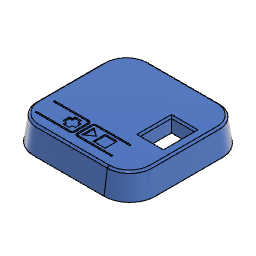
Abdeckung (Autodesk Fusion 360 design; units mm, degrees)
Autodesk Fusion 360 part; units mm, degrees
ref_plane "Arbeitsebene1" through (35.3452, 7.7218, 7.3701) normal (0, 0, 1) x (1, 0, 0)
sketch "Skizze1" plane through (35.3452, 7.7218, 7.3701) normal (0, 0, 1) x (1, 0, 0)
  line L0 (-56.34, -21.7733) -> (-56.34, 68.7267)
  arc A0 (-56.34, -21.7733) -> (-41.34, -36.7733) centre (-41.34, -21.7733) ccw
  line L1 (-0.34, -36.7733) -> (-41.34, -36.7733)
  arc A1 (-0.34, -36.7733) -> (14.66, -21.7733) centre (-0.34, -21.7733) ccw
  line L2 (14.66, 68.7267) -> (14.66, -21.7733)
  line L3 (12.66, 17.2267) -> (12.66, -21.7733)
  arc A2 (-0.34, -34.7733) -> (12.66, -21.7733) centre (-0.34, -21.7733) ccw
  line L4 (-0.34, -34.7733) -> (-41.34, -34.7733)
  arc A3 (-54.34, -21.7733) -> (-41.34, -34.7733) centre (-41.34, -21.7733) ccw
  line L5 (-54.34, -21.7733) -> (-54.34, 17.2267)
  line L6 (-41.34, 30.2267) -> (-0.34, 30.2267)
  circle A4 centre (-20.84, -2.2733) radius 32.5
  arc A5 (-41.34, 30.2267) -> (-54.34, 17.2267) centre (-41.34, 17.2267) ccw
  arc A6 (12.66, 17.2267) -> (-0.34, 30.2267) centre (-0.34, 17.2267) ccw
  dimension "d140" = 13
  dimension "d141" = 13
  constraint perpendicular L3 L6
  constraint tangent L6 A4
  constraint parallel L2 L3
  constraint concentric A1 A2
  constraint parallel L1 L4
  constraint concentric A0 A3
  constraint parallel L0 L5
  constraint tangent L4 A3
  constraint tangent L3 A2
  constraint tangent A2 L4
  constraint tangent A3 L5
  constraint tangent L5 A5
  constraint tangent L6 A5
  constraint tangent L4 A4
  constraint tangent L6 A6
  constraint tangent L3 A6
  measures "d140" radius of A5
  measures "d141" radius of A6
sketch "Skizze3" plane through (0, 0, -6.9849) normal (0, 0, 1) x (-1, 0, 0)
  circle A0 centre (-14.5052, -5.4485) radius 32.5
  circle A1 centre (-14.5052, -63.9485) radius 21.5
  arc A2 (-35.0052, 29.0515) -> (-50.0052, 14.0515) centre (-35.0052, 14.0515) ccw
  line L0 (-50.0052, 14.0515) -> (-50.0052, -76.4485)
  arc A3 (-50.0052, -76.4485) -> (-35.0052, -91.4485) centre (-35.0052, -76.4485) ccw
  line L1 (-35.0052, -91.4485) -> (5.9948, -91.4485)
  arc A4 (5.9948, -91.4485) -> (20.9948, -76.4485) centre (5.9948, -76.4485) ccw
  line L2 (20.9948, -76.4485) -> (20.9948, 14.0515)
  arc A5 (20.9948, 14.0515) -> (5.9948, 29.0515) centre (5.9948, 14.0515) ccw
  line L3 (5.9948, 29.0515) -> (-35.0052, 29.0515)
  arc A6 (20.9948, 14.0515) -> (5.9948, 29.0515) centre (5.9948, 14.0515) ccw
  line L4 (-35.0052, 29.0515) -> (5.9948, 29.0515)
  arc A7 (-35.0052, 29.0515) -> (-50.0052, 14.0515) centre (-35.0052, 14.0515) ccw
  line L5 (-50.0052, -76.4485) -> (-50.0052, 14.0515)
  line L6 (20.9948, 14.0515) -> (20.9948, -76.4485)
  line L7 (5.9948, -39.9485) -> (-35.0052, -39.9485)
  arc A8 (5.9948, -39.9485) -> (20.9607, -23.9379) centre (5.9948, -24.9485) ccw
  arc A9 (-50.0052, -24.9485) -> (-35.0052, -39.9485) centre (-35.0052, -24.9485) ccw
  arc A10 (5.9948, -37.9485) -> (18.9948, -24.9485) centre (5.9948, -24.9485) ccw
  constraint perpendicular L0 L7
  constraint tangent L2 A8
  constraint tangent L5 A9
  constraint tangent L7 A8
  constraint tangent L7 A9
  constraint equal A8 A9
  constraint concentric A8 A10
  constraint coincident L5 A9.start
loft "Erhebung1" add profiles "Skizze3", "Skizze1" section 1 contours A2 L0 L2 A5 L3 A6 L4 A7 L5 L6 L7 A8 A9 section 2
sketch "Skizze4" plane through (0, 0, -6.9849) normal (0, 0, -1) x (1, 0, 0)
  spline S0 degree 3 poles (35.0052, 29.0515) (36.8795, 29.0515) (38.8639, 28.6884) (40.741, 27.9116) (42.1372, 27.3338) (43.4713, 26.5301) (44.6549, 25.5356) (46.3943, 24.074) (47.7962, 22.1974) (48.704, 20.1624) (49.5899, 18.1766) (50.0052, 16.0511) (50.0052, 14.0515) (50.0052, 1.0515) (50.0052, -11.9485) (50.0052, -24.9485) (50.0052, -26.8227) (49.6421, -28.8072) (48.8653, -30.6842) (48.2875, -32.0805) (47.4838, -33.4146) (46.4893, -34.5981) (45.0277, -36.3376) (43.1511, -37.7395) (41.1162, -38.6473) (39.1303, -39.5331) (37.0049, -39.9485) (35.0052, -39.9485) (21.3386, -39.9485) (7.6719, -39.9485) (-5.9948, -39.9485) (-7.869, -39.9485) (-9.8534, -39.5853) (-11.7305, -38.8085) (-13.1268, -38.2307) (-14.4609, -37.4271) (-15.6444, -36.4326) (-17.3839, -34.971) (-18.7858, -33.0943) (-19.6935, -31.0594) (-20.5794, -29.0736) (-20.9948, -26.9481) (-20.9948, -24.9485) (-20.9948, -11.9485) (-20.9948, 1.0515) (-20.9948, 14.0515) (-20.9948, 15.9258) (-20.6316, 17.9102) (-19.8548, 19.7872) (-19.277, 21.1835) (-18.4733, 22.5176) (-17.4789, 23.7011) (-16.0173, 25.4406) (-14.1406, 26.8425) (-12.1057, 27.7503) (-10.1199, 28.6362) (-7.9944, 29.0515) (-5.9948, 29.0515) (7.6719, 29.0515) (21.3386, 29.0515) (35.0052, 29.0515) knots 0 0 0 0 0.02269 0.02269 0.02269 0.039568 0.039568 0.039568 0.064375 0.064375 0.064375 0.088583 0.088583 0.088583 0.245965 0.245965 0.245965 0.268655 0.268655 0.268655 0.285533 0.285533 0.285533 0.31034 0.31034 0.31034 0.334548 0.334548 0.334548 0.5 0.5 0.5 0.52269 0.52269 0.52269 0.539568 0.539568 0.539568 0.564375 0.564375 0.564375 0.588583 0.588583 0.588583 0.745965 0.745965 0.745965 0.768655 0.768655 0.768655 0.785533 0.785533 0.785533 0.81034 0.81034 0.81034 0.834548 0.834548 0.834548 1 1 1 1
  circle A0 centre (14.5052, -5.4485) radius 32.5
extrude "Extrusion1" cut sketch "Skizze4" against normal blind 12 contours A0
sketch "Skizze5" plane through (0, 0, 7.3701) normal (0, 0, 1) x (-1, 0, 0)
  spline S0 degree 3 poles (-35.0052, 27.0515) (-36.7488, 27.0515) (-38.4915, 26.6961) (-40.0958, 26.0134) (-41.2892, 25.5055) (-42.4058, 24.8178) (-43.3964, 23.9807) (-44.8523, 22.7503) (-46.0324, 21.1954) (-46.8257, 19.4622) (-47.6, 17.7708) (-48.0052, 15.9117) (-48.0052, 14.0515) (-48.0052, 1.9582) (-48.0052, -12.8552) (-48.0052, -24.9485) (-48.0052, -26.692) (-47.6498, -28.4348) (-46.9671, -30.0391) (-46.4592, -31.2324) (-45.7716, -32.3491) (-44.9344, -33.3396) (-43.704, -34.7955) (-42.1491, -35.9756) (-40.4159, -36.769) (-38.7245, -37.5432) (-36.8654, -37.9485) (-35.0052, -37.9485) (-22.2917, -37.9485) (-6.7187, -37.9485) (5.9948, -37.9485) (7.7383, -37.9485) (9.481, -37.5931) (11.0853, -36.9103) (12.2787, -36.4025) (13.3953, -35.7148) (14.3859, -34.8777) (15.8418, -33.6473) (17.0219, -32.0924) (17.8153, -30.3592) (18.5895, -28.6678) (18.9948, -26.8087) (18.9948, -24.9485) (18.9948, -12.8552) (18.9948, 1.9582) (18.9948, 14.0515) (18.9948, 15.795) (18.6394, 17.5378) (17.9566, 19.1421) (17.4488, 20.3354) (16.7611, 21.4521) (15.924, 22.4427) (14.6936, 23.8986) (13.1387, 25.0787) (11.4054, 25.872) (9.7141, 26.6462) (7.8549, 27.0515) (5.9948, 27.0515) (-6.7187, 27.0515) (-22.2917, 27.0515) (-35.0052, 27.0515) knots 0 0 0 0 0.02269 0.02269 0.02269 0.039568 0.039568 0.039568 0.064375 0.064375 0.064375 0.088583 0.088583 0.088583 0.245965 0.245965 0.245965 0.268655 0.268655 0.268655 0.285533 0.285533 0.285533 0.31034 0.31034 0.31034 0.334548 0.334548 0.334548 0.5 0.5 0.5 0.52269 0.52269 0.52269 0.539568 0.539568 0.539568 0.564375 0.564375 0.564375 0.588583 0.588583 0.588583 0.745965 0.745965 0.745965 0.768655 0.768655 0.768655 0.785533 0.785533 0.785533 0.81034 0.81034 0.81034 0.834548 0.834548 0.834548 1 1 1 1
  line L0 (-41.6202, -16.3468) -> (-29.0702, -16.3468)
  line L1 (-29.0702, -16.3468) -> (-29.0702, 0.9032)
  line L2 (-29.0702, 0.9032) -> (-41.6202, 0.9032)
  line L3 (-41.6202, 0.9032) -> (-41.6202, -16.3468)
  line L4 (-33.512, -14.2079) -> (-33.069, -14.7358)
  line L5 (-33.069, -14.7358) -> (-33.4529, -15.0579)
  line L6 (-33.4529, -15.0579) -> (-39.8251, -15.0579)
  line L7 (-39.8251, -15.0579) -> (-40.0801, -14.7541)
  line L8 (-40.0801, -14.7541) -> (-39.4292, -14.2079)
  line L9 (-39.4292, -14.2079) -> (-33.512, -14.2079)
  line L10 (-39.6216, -13.9781) -> (-40.2727, -14.5245)
  line L11 (-40.2727, -14.5245) -> (-40.5275, -14.2209)
  line L12 (-40.5275, -14.2209) -> (-39.4684, -8.2142)
  line L13 (-39.4684, -8.2142) -> (-38.976, -7.8695)
  line L14 (-38.976, -7.8695) -> (-38.6313, -8.3618)
  line L15 (-38.6313, -8.3618) -> (-39.6216, -13.9781)
  line L16 (-39.2687, -7.0817) -> (-38.3065, -1.625)
  line L17 (-38.3065, -1.625) -> (-37.9226, -1.3029)
  line L18 (-37.9226, -1.3029) -> (-37.9169, -1.3098)
  line L19 (-37.9169, -1.3098) -> (-37.4797, -1.8308)
  line L20 (-37.4797, -1.8308) -> (-38.4316, -7.2293)
  line L21 (-38.4316, -7.2293) -> (-38.924, -7.5741)
  line L22 (-38.924, -7.5741) -> (-39.2687, -7.0817)
  circle A0 centre (-39.5952, -1.6629) radius 0.875
  line L23 (-31.1397, -1.8673) -> (-30.4891, -1.3214)
  line L24 (-30.4891, -1.3214) -> (-30.234, -1.6255)
  line L25 (-30.234, -1.6255) -> (-31.2221, -7.2293)
  line L26 (-31.2221, -7.2293) -> (-31.7144, -7.5741)
  line L27 (-31.7144, -7.5741) -> (-32.0592, -7.0817)
  line L28 (-32.0592, -7.0817) -> (-31.1397, -1.8673)
  line L29 (-32.133, -7.5003) -> (-32.1322, -7.5004)
  line L30 (-32.1322, -7.5004) -> (-32.0106, -7.6742)
  line L31 (-32.0106, -7.6742) -> (-32.1843, -7.7958)
  line L32 (-32.1843, -7.7958) -> (-32.1851, -7.7957)
  line L33 (-32.1851, -7.7957) -> (-32.1852, -7.7964)
  line L34 (-32.1852, -7.7964) -> (-32.6855, -8.1468)
  line L35 (-32.6855, -8.1468) -> (-38.4157, -8.1468)
  line L36 (-38.4157, -8.1468) -> (-38.5576, -7.944)
  line L37 (-38.5576, -7.944) -> (-38.5575, -7.9433)
  line L38 (-38.5575, -7.9433) -> (-38.5582, -7.9432)
  line L39 (-38.5582, -7.9432) -> (-38.6799, -7.7694)
  line L40 (-38.6799, -7.7694) -> (-38.5061, -7.6477)
  line L41 (-38.5061, -7.6477) -> (-38.5054, -7.6479)
  line L42 (-38.5054, -7.6479) -> (-38.5053, -7.6471)
  line L43 (-38.5053, -7.6471) -> (-38.0049, -7.2968)
  line L44 (-38.0049, -7.2968) -> (-32.2748, -7.2968)
  line L45 (-32.2748, -7.2968) -> (-32.1328, -7.4995)
  line L46 (-32.1328, -7.4995) -> (-32.133, -7.5003)
  line L47 (-31.4218, -8.3618) -> (-32.4548, -14.2204)
  line L48 (-32.4548, -14.2204) -> (-32.8392, -14.543)
  line L49 (-32.8392, -14.543) -> (-33.2818, -14.0156)
  line L50 (-33.2818, -14.0156) -> (-32.2589, -8.2142)
  line L51 (-32.2589, -8.2142) -> (-31.7665, -7.8695)
  line L52 (-31.7665, -7.8695) -> (-31.4218, -8.3618)
  line L53 (-37.2503, -1.6379) -> (-37.6931, -1.1103)
  line L54 (-37.6931, -1.1103) -> (-37.3089, -0.7879)
  line L55 (-37.3089, -0.7879) -> (-30.9368, -0.7879)
  line L56 (-30.9368, -0.7879) -> (-30.682, -1.0916)
  line L57 (-30.682, -1.0916) -> (-31.3331, -1.6379)
  line L58 (-31.3331, -1.6379) -> (-37.2503, -1.6379)
  circle A1 centre (-39.5952, -1.6629) radius 0.875
  line L59 (-37.9226, -1.3029) -> (-38.3065, -1.625)
  line L60 (-38.3065, -1.625) -> (-39.2687, -7.0817)
  line L61 (-39.2687, -7.0817) -> (-38.924, -7.5741)
  line L62 (-38.924, -7.5741) -> (-38.4316, -7.2293)
  line L63 (-38.4316, -7.2293) -> (-37.4797, -1.8308)
  line L64 (-37.4797, -1.8308) -> (-37.9169, -1.3098)
  line L65 (-37.9169, -1.3098) -> (-37.9226, -1.3029)
  line L66 (-37.3089, -0.7879) -> (-37.6931, -1.1103)
  line L67 (-37.6931, -1.1103) -> (-37.2503, -1.6379)
  line L68 (-37.2503, -1.6379) -> (-31.3331, -1.6379)
  line L69 (-31.3331, -1.6379) -> (-30.682, -1.0916)
  line L70 (-30.682, -1.0916) -> (-30.9368, -0.7879)
  line L71 (-30.9368, -0.7879) -> (-37.3089, -0.7879)
  line L72 (-30.234, -1.6255) -> (-30.4891, -1.3214)
  line L73 (-30.4891, -1.3214) -> (-31.1397, -1.8673)
  line L74 (-31.1397, -1.8673) -> (-32.0592, -7.0817)
  line L75 (-32.0592, -7.0817) -> (-31.7144, -7.5741)
  line L76 (-31.7144, -7.5741) -> (-31.2221, -7.2293)
  line L77 (-31.2221, -7.2293) -> (-30.234, -1.6255)
  line L78 (-32.1851, -7.7957) -> (-32.1843, -7.7958)
  line L79 (-32.1843, -7.7958) -> (-32.0106, -7.6742)
  line L80 (-32.0106, -7.6742) -> (-32.1322, -7.5004)
  line L81 (-32.1322, -7.5004) -> (-32.133, -7.5003)
  line L82 (-32.133, -7.5003) -> (-32.1328, -7.4995)
  line L83 (-32.1328, -7.4995) -> (-32.2748, -7.2968)
  line L84 (-32.2748, -7.2968) -> (-38.0049, -7.2968)
  line L85 (-38.0049, -7.2968) -> (-38.5053, -7.6471)
  line L86 (-38.5053, -7.6471) -> (-38.5054, -7.6479)
  line L87 (-38.5054, -7.6479) -> (-38.5061, -7.6477)
  line L88 (-38.5061, -7.6477) -> (-38.6799, -7.7694)
  line L89 (-38.6799, -7.7694) -> (-38.5582, -7.9432)
  line L90 (-38.5582, -7.9432) -> (-38.5575, -7.9433)
  line L91 (-38.5575, -7.9433) -> (-38.5576, -7.944)
  line L92 (-38.5576, -7.944) -> (-38.4157, -8.1468)
  line L93 (-38.4157, -8.1468) -> (-32.6855, -8.1468)
  line L94 (-32.6855, -8.1468) -> (-32.1852, -7.7964)
  line L95 (-32.1852, -7.7964) -> (-32.1851, -7.7957)
  line L96 (-32.8392, -14.543) -> (-32.4548, -14.2204)
  line L97 (-32.4548, -14.2204) -> (-31.4218, -8.3618)
  line L98 (-31.4218, -8.3618) -> (-31.7665, -7.8695)
  line L99 (-31.7665, -7.8695) -> (-32.2589, -8.2142)
  line L100 (-32.2589, -8.2142) -> (-33.2818, -14.0156)
  line L101 (-33.2818, -14.0156) -> (-32.8392, -14.543)
  line L102 (-33.4529, -15.0579) -> (-33.069, -14.7358)
  line L103 (-33.069, -14.7358) -> (-33.512, -14.2079)
  line L104 (-33.512, -14.2079) -> (-39.4292, -14.2079)
  line L105 (-39.4292, -14.2079) -> (-40.0801, -14.7541)
  line L106 (-40.0801, -14.7541) -> (-39.8251, -15.0579)
  line L107 (-39.8251, -15.0579) -> (-33.4529, -15.0579)
  line L108 (-40.5275, -14.2209) -> (-40.2727, -14.5245)
  line L109 (-40.2727, -14.5245) -> (-39.6216, -13.9781)
  line L110 (-39.6216, -13.9781) -> (-38.6313, -8.3618)
  line L111 (-38.6313, -8.3618) -> (-38.976, -7.8695)
  line L112 (-38.976, -7.8695) -> (-39.4684, -8.2142)
  line L113 (-39.4684, -8.2142) -> (-40.5275, -14.2209)
  line L114 (-28.5702, -16.8468) -> (-42.1202, -16.8468)
  line L115 (-42.1202, -16.8468) -> (-42.1202, 1.4032)
  line L116 (-42.1202, 1.4032) -> (-28.5702, 1.4032)
  line L117 (-28.5702, 1.4032) -> (-28.5702, -16.8468)
  dimension "d144" = 0.5
  dimension "d145" = 0.5
  dimension "d146" = 0.5
  dimension "d147" = 0.5
  constraint horizontal L114
  constraint vertical L115
  constraint horizontal L116
  constraint vertical L117
  measures "d144" distance of L1 L117
  measures "d145" distance of L3 L115
  measures "d146" distance of L0 L114
  measures "d147" distance of L2 L116
extrude "Extrusion2" cut sketch "Skizze5" against normal up to surface (2.355 mm away) contours L0 L1 L2 L3 | L4 L5 L6 L7 L8 L9 L102 L103 L104 L105 L106 L107 | L10 L11 L12 L13 L14 L15 L108 L109 L110 L111 L112 L113 | L16 L17 L18 L19 L20 L21 L22 L59 L60 L61 L62 L63 L64 L65 | A0 A1 | L23 L24 L25 L26 L27 L28 L72 L73 L74 L75 L76 L77 | L30 L31 L34 L35 L36 L39 L40 L43 L44 L45 L79 L80 L83 L84 L85 L88 L89 L92 L93 L94 | L47 L48 L49 L50 L51 L52 L96 L97 L98 L99 L100 L101 | L53 L54 L55 L56 L57 L58 L66 L67 L68 L69 L70 L71 | L114 L115 L116 L117
sketch "Skizze6" plane through (0, 0, 5.0151) normal (0, 0, -1) x (1, 0, 0)
  line L0 (28.5702, -16.8468) -> (28.5702, 1.4032)
  line L1 (28.5702, 1.4032) -> (42.1202, 1.4032)
  line L2 (42.1202, 1.4032) -> (42.1202, -16.8468)
  line L3 (42.1202, -16.8468) -> (28.5702, -16.8468)
  circle A0 centre (14.5052, -5.4485) radius 32.5
  circle A1 centre (3.0052, 15.1382) radius 1.75
  circle A2 centre (14.5052, 15.1382) radius 1.75
  circle A3 centre (14.5052, 15.1382) radius 1.75
  line L4 (11.3552, 18.2882) -> (17.6552, 18.2882)
  line L5 (17.6552, 18.2882) -> (17.6552, 11.9882)
  line L6 (17.6552, 11.9882) -> (11.3552, 11.9882)
  line L7 (11.3552, 11.9882) -> (11.3552, 18.2882)
  circle A4 centre (3.0052, 15.1382) radius 1.75
  line L8 (-0.1448, 18.2882) -> (6.1552, 18.2882)
  line L9 (6.1552, 18.2882) -> (6.1552, 11.9882)
  line L10 (6.1552, 11.9882) -> (-0.1448, 11.9882)
  line L11 (-0.1448, 11.9882) -> (-0.1448, 18.2882)
  line L12 (6.4052, 9.3882) -> (-13.5948, 9.3882)
  line L13 (-13.5948, 20.8882) -> (6.4052, 20.8882)
  line L14 (8.1552, 19.1382) -> (8.1552, 11.1382)
  line L15 (31.1052, 9.3882) -> (11.1052, 9.3882)
  line L16 (9.3552, 11.1382) -> (9.3552, 19.1382)
  line L17 (11.1052, 20.8882) -> (31.1052, 20.8882)
  line L18 (6.4052, 10.1382) -> (-13.5948, 10.1382)
  line L19 (-13.5948, 20.1382) -> (6.4052, 20.1382)
  line L20 (7.4052, 19.1382) -> (7.4052, 11.1382)
  line L21 (31.1052, 10.1382) -> (11.1052, 10.1382)
  line L22 (10.1052, 11.1382) -> (10.1052, 19.1382)
  line L23 (11.1052, 20.1382) -> (31.1052, 20.1382)
  arc A5 (7.4052, 19.1382) -> (6.4052, 20.1382) centre (6.4052, 19.1382) ccw
  arc A6 (6.4052, 10.1382) -> (7.4052, 11.1382) centre (6.4052, 11.1382) ccw
  arc A7 (11.1052, 20.1382) -> (10.1052, 19.1382) centre (11.1052, 19.1382) ccw
  arc A8 (10.1052, 11.1382) -> (11.1052, 10.1382) centre (11.1052, 11.1382) ccw
  arc A9 (8.1552, 19.1382) -> (6.4052, 20.8882) centre (6.4052, 19.1382) ccw
  arc A10 (6.4052, 9.3882) -> (8.1552, 11.1382) centre (6.4052, 11.1382) ccw
  arc A11 (11.1052, 20.8882) -> (9.3552, 19.1382) centre (11.1052, 19.1382) ccw
  arc A12 (9.3552, 11.1382) -> (11.1052, 9.3882) centre (11.1052, 11.1382) ccw
  line L24 (-13.5948, 9.3882) -> (-13.5948, 10.1382)
  line L25 (-13.5948, 20.1382) -> (-13.5948, 20.8882)
  line L26 (31.1052, 20.8882) -> (31.1052, 20.1382)
  line L27 (31.1052, 10.1382) -> (31.1052, 9.3882)
  point P0 (3.0052, 15.1382)
  point P1 (14.5052, 15.1382)
  dimension "d154" = 1
  dimension "d155" = 1
  dimension "d157" = 0.75
  dimension "d158" = 1
  dimension "d159" = 1
  dimension "d160" = 0.75
  dimension "d208" = 1.25
  dimension "d209" = 1.25
  dimension "d210" = 10
  dimension "d211" = 5
  dimension "d217" = 20
  constraint horizontal L12
  constraint perpendicular L12 L24
  constraint parallel L12 L13
  constraint parallel L14 L24
  constraint coincident P0 A1.centre
  constraint horizontal L15
  constraint perpendicular L15 L16
  constraint parallel L15 L17
  constraint parallel L16 L26
  constraint coincident P1 A2.centre
  constraint parallel L12 L18
  constraint parallel L13 L19
  constraint parallel L14 L20
  constraint tangent L19 A5
  constraint tangent L20 A5
  constraint tangent L18 A6
  constraint tangent L20 A6
  constraint parallel L15 L21
  constraint parallel L16 L22
  constraint parallel L17 L23
  constraint tangent L23 A7
  constraint tangent L22 A7
  constraint tangent L22 A8
  constraint tangent L21 A8
  constraint coincident L19.start L24
  constraint coincident L21.start L26
  constraint tangent L13 A9
  constraint tangent L14 A9
  constraint concentric A5 A9
  constraint tangent L12 A10
  constraint tangent L14 A10
  constraint tangent L16 A11
  constraint tangent L17 A11
  constraint tangent L16 A12
  constraint tangent L15 A12
  constraint concentric A6 A10
  constraint concentric A7 A11
  constraint concentric A8 A12
  constraint horizontal L13.end L17.start
  constraint horizontal L12.start L15.end
  constraint collinear L24 L25
  constraint collinear L26 L27
  constraint equal L13 L17
  measures "d154" radius of A5
  measures "d155" radius of A6
  measures "d157" distance of L13 L19
  measures "d158" radius of A7
  measures "d159" radius of A8
  measures "d160" distance of L17 L23
  measures "d208" distance of L9 L20
  measures "d209" distance of L7 L22
  measures "d210" distance of L21 L23
  measures "d211" vertical distance of P1 L23.end
  measures "d217" distance of L21.start L21.end
extrude "Extrusion3" cut sketch "Skizze6" against normal up to surface (2.355 mm away) contours A0 L12 L13 L14 L18 L19 L20 A5 A6 A9 A10 L24 | A0 L13 L19 L25 | L15 L16 L17 L21 L22 L23 A7 A8 A11 A12 L26 L27 picked at (-0.2614, 9.8882)
sketch "Skizze7" plane through (0, 0, 5.0151) normal (0, 0, -1) x (1, 0, 0)
  arc A0 (7.4052, 19.1382) -> (6.4052, 20.1382) centre (6.4052, 19.1382) ccw
  line L0 (6.4052, 20.1382) -> (-5.534, 20.1382)
  line L1 (-4.5376, 20.8882) -> (6.4052, 20.8882)
  arc A1 (8.1552, 19.1382) -> (6.4052, 20.8882) centre (6.4052, 19.1382) ccw
  line L2 (8.1552, 19.1382) -> (8.1552, 11.1382)
  arc A2 (6.4052, 9.3882) -> (8.1552, 11.1382) centre (6.4052, 11.1382) ccw
  line L3 (6.4052, 9.3882) -> (-13.5948, 9.3882)
  line L4 (-13.5948, 9.3882) -> (-13.5948, 10.1382)
  line L5 (-13.5948, 10.1382) -> (6.4052, 10.1382)
  arc A3 (6.4052, 10.1382) -> (7.4052, 11.1382) centre (6.4052, 11.1382) ccw
  line L6 (7.4052, 11.1382) -> (7.4052, 19.1382)
  line L7 (10.1052, 19.1382) -> (10.1052, 11.1382)
  arc A4 (10.1052, 11.1382) -> (11.1052, 10.1382) centre (11.1052, 11.1382) ccw
  line L8 (11.1052, 10.1382) -> (31.1052, 10.1382)
  line L9 (31.1052, 10.1382) -> (31.1052, 9.3882)
  line L10 (31.1052, 9.3882) -> (11.1052, 9.3882)
  arc A5 (9.3552, 11.1382) -> (11.1052, 9.3882) centre (11.1052, 11.1382) ccw
  line L11 (9.3552, 11.1382) -> (9.3552, 19.1382)
  arc A6 (11.1052, 20.8882) -> (9.3552, 19.1382) centre (11.1052, 19.1382) ccw
  line L12 (11.1052, 20.8882) -> (31.1052, 20.8882)
  line L13 (31.1052, 20.8882) -> (31.1052, 20.1382)
  line L14 (31.1052, 20.1382) -> (11.1052, 20.1382)
  arc A7 (11.1052, 20.1382) -> (10.1052, 19.1382) centre (11.1052, 19.1382) ccw
  line L15 (28.5702, -16.8468) -> (28.5702, 1.4032)
  line L16 (28.5702, 1.4032) -> (42.1202, 1.4032)
  line L17 (42.1202, 1.4032) -> (42.1202, -16.8468)
  line L18 (42.1202, -16.8468) -> (28.5702, -16.8468)
  line L19 (-13.5948, 20.1382) -> (-11.5948, 20.1382)
  line L20 (-11.5948, 20.1382) -> (-11.5948, 10.1382)
  line L21 (-11.5948, 10.1382) -> (-13.5948, 10.1382)
  line L22 (-13.5948, 10.1382) -> (-13.5948, 20.1382)
  line L23 (31.1052, 20.1382) -> (29.1052, 20.1382)
  line L24 (29.1052, 20.1382) -> (29.1052, 10.1382)
  line L25 (29.1052, 10.1382) -> (31.1052, 10.1382)
  line L26 (31.1052, 10.1382) -> (31.1052, 20.1382)
  arc A8 (-5.534, 20.1382) -> (-4.5376, 20.8882) centre (14.5052, -5.4485) ccw
  point P0 (-13.5948, 20.1382)
  dimension "d167" = 2
  dimension "d168" = 2
  constraint horizontal L19
  constraint vertical L20
  constraint horizontal L21
  constraint vertical L22
  constraint coincident L5 L20.end
  constraint horizontal L23
  constraint vertical L24
  constraint horizontal L25
  constraint vertical L26
  constraint coincident L8 L24.end
  constraint coincident L13.end L14.start
  constraint coincident P0 L19.start
  measures "d167" distance of P0 L19.end
  measures "d168" distance of L13.end L23.end
sketch "Skizze12" plane through (0, 0, 5.0151) normal (0, 0, -1) x (1, 0, 0)
  line L0 (-13.5948, 9.3882) -> (-13.5948, 10.1382)
  arc A0 (-5.534, 20.1382) -> (-4.5376, 20.8882) centre (14.5052, -5.4485) ccw
  line L1 (-4.5376, 20.8882) -> (6.4052, 20.8882)
  arc A1 (8.1552, 19.1382) -> (6.4052, 20.8882) centre (6.4052, 19.1382) ccw
  line L2 (8.1552, 19.1382) -> (8.1552, 11.1382)
  arc A2 (6.4052, 9.3882) -> (8.1552, 11.1382) centre (6.4052, 11.1382) ccw
  line L3 (6.4052, 9.3882) -> (-13.5948, 9.3882)
  line L4 (28.5702, -16.8468) -> (28.5702, 1.4032)
  line L5 (28.5702, 1.4032) -> (42.1202, 1.4032)
  line L6 (42.1202, 1.4032) -> (42.1202, -16.8468)
  line L7 (42.1202, -16.8468) -> (28.5702, -16.8468)
  line L8 (31.1052, 20.8882) -> (31.1052, 20.1382)
  line L9 (31.1052, 9.3882) -> (11.1052, 9.3882)
  arc A3 (9.3552, 11.1382) -> (11.1052, 9.3882) centre (11.1052, 11.1382) ccw
  line L10 (9.3552, 11.1382) -> (9.3552, 19.1382)
  arc A4 (11.1052, 20.8882) -> (9.3552, 19.1382) centre (11.1052, 19.1382) ccw
  line L11 (11.1052, 20.8882) -> (31.1052, 20.8882)
  arc A5 (-5.534, 20.1382) -> (-4.5376, 20.8882) centre (14.5052, -5.4485) ccw
  arc A6 (-4.5376, 20.8882) -> (-5.534, 20.1382) centre (14.5052, -5.4485) ccw
  arc A7 (-5.534, 20.1382) -> (-4.5376, 20.8882) centre (14.5052, -5.4485) ccw
  arc A8 (-4.5376, 20.8882) -> (-5.534, 20.1382) centre (14.5052, -5.4485) ccw
  line L12 (-13.5948, 9.3882) -> (-13.5948, 10.1382)
  line L13 (-13.5948, 20.1382) -> (-13.5948, 20.8882)
  line L14 (-13.5948, 20.8882) -> (-4.5376, 20.8882)
  line L15 (-13.5948, 10.1382) -> (6.4052, 10.1382)
  arc A9 (6.4052, 10.1382) -> (7.4052, 11.1382) centre (6.4052, 11.1382) ccw
  line L16 (7.4052, 11.1382) -> (7.4052, 19.1382)
  arc A10 (7.4052, 19.1382) -> (6.4052, 20.1382) centre (6.4052, 19.1382) ccw
  line L17 (6.4052, 20.1382) -> (-5.534, 20.1382)
  line L18 (31.1052, 20.1382) -> (11.1052, 20.1382)
  arc A11 (11.1052, 20.1382) -> (10.1052, 19.1382) centre (11.1052, 19.1382) ccw
  line L19 (10.1052, 19.1382) -> (10.1052, 11.1382)
  arc A12 (10.1052, 11.1382) -> (11.1052, 10.1382) centre (11.1052, 11.1382) ccw
  line L20 (11.1052, 10.1382) -> (31.1052, 10.1382)
  line L21 (31.1052, 10.1382) -> (31.1052, 9.3882)
  line L22 (-13.5948, 20.1382) -> (-13.5948, 10.1382)
  constraint coincident L13.end L14.start
  constraint coincident A0.end L1.start
  constraint coincident L13.start L22.start
  constraint coincident L0.end L12.end
extrude "Extrusion11" cut sketch "Skizze12" along normal blind 1.5 contours L0 A0 L1 A1 L2 A2 L3 A5 A7 L12 L22 | L0 L1 A1 L2 A2 L3 A6 A8 L12 L15 A9 L16 A10 L17 | A0 A5 A7 L15 A9 L16 A10 L17 L22 | A0 A5 A6 A7 A8 L13 L14 L22 | L4 L5 L6 L7 | L8 L9 A3 L10 A4 L11 L18 A11 L19 A12 L20 L21
sketch "Skizze13" plane through (0, 0, 5.0151) normal (0, 0, -1) x (1, 0, 0)
  line L0 (-4.5376, 20.8882) -> (6.4052, 20.8882)
  arc A0 (8.1552, 19.1382) -> (6.4052, 20.8882) centre (6.4052, 19.1382) ccw
  line L1 (8.1552, 19.1382) -> (8.1552, 11.1382)
  arc A1 (6.4052, 9.3882) -> (8.1552, 11.1382) centre (6.4052, 11.1382) ccw
  line L2 (6.4052, 9.3882) -> (-13.5948, 9.3882)
  line L3 (-13.5948, 9.3882) -> (-13.5948, 10.1382)
  line L4 (-13.5948, 10.1382) -> (6.4052, 10.1382)
  arc A2 (6.4052, 10.1382) -> (7.4052, 11.1382) centre (6.4052, 11.1382) ccw
  line L5 (7.4052, 11.1382) -> (7.4052, 19.1382)
  arc A3 (7.4052, 19.1382) -> (6.4052, 20.1382) centre (6.4052, 19.1382) ccw
  line L6 (6.4052, 20.1382) -> (-13.5948, 20.1382)
  line L7 (-13.5948, 20.1382) -> (-13.5948, 10.8806)
  arc A4 (-13.5948, 10.8806) -> (-4.5376, 20.8882) centre (14.5052, -5.4485) ccw
  line L8 (28.5702, -16.8468) -> (28.5702, 1.4032)
  line L9 (28.5702, 1.4032) -> (42.1202, 1.4032)
  line L10 (42.1202, 1.4032) -> (42.1202, -16.8468)
  line L11 (42.1202, -16.8468) -> (28.5702, -16.8468)
  arc A5 (9.3552, 11.1382) -> (11.1052, 9.3882) centre (11.1052, 11.1382) ccw
  line L12 (9.3552, 11.1382) -> (9.3552, 19.1382)
  arc A6 (11.1052, 20.8882) -> (9.3552, 19.1382) centre (11.1052, 19.1382) ccw
  line L13 (11.1052, 20.8882) -> (31.1052, 20.8882)
  line L14 (31.1052, 20.8882) -> (31.1052, 20.1382)
  line L15 (31.1052, 20.1382) -> (11.1052, 20.1382)
  arc A7 (11.1052, 20.1382) -> (10.1052, 19.1382) centre (11.1052, 19.1382) ccw
  line L16 (10.1052, 19.1382) -> (10.1052, 11.1382)
  arc A8 (10.1052, 11.1382) -> (11.1052, 10.1382) centre (11.1052, 11.1382) ccw
  line L17 (11.1052, 10.1382) -> (31.1052, 10.1382)
  line L18 (31.1052, 10.1382) -> (31.1052, 9.3882)
  line L19 (31.1052, 9.3882) -> (11.1052, 9.3882)
  line L20 (7.4052, 11.1382) -> (7.4052, 19.1382)
  arc A9 (7.4052, 19.1382) -> (6.4052, 20.1382) centre (6.4052, 19.1382) ccw
  line L21 (-13.5948, 20.1382) -> (6.4052, 20.1382)
  line L22 (-13.5948, 10.1382) -> (6.4052, 10.1382)
  arc A10 (6.4052, 10.1382) -> (7.4052, 11.1382) centre (6.4052, 11.1382) ccw
  line L23 (31.1052, 20.1382) -> (11.1052, 20.1382)
  arc A11 (11.1052, 20.1382) -> (10.1052, 19.1382) centre (11.1052, 19.1382) ccw
  line L24 (10.1052, 19.1382) -> (10.1052, 11.1382)
  arc A12 (10.1052, 11.1382) -> (11.1052, 10.1382) centre (11.1052, 11.1382) ccw
  line L25 (11.1052, 10.1382) -> (31.1052, 10.1382)
  line L26 (-2.5948, 20.1382) -> (-2.5948, 10.1382)
  line L27 (20.1052, 20.1382) -> (20.1052, 10.1382)
  dimension "d222" = 10
  dimension "d223" = 10
  constraint coincident L6 L26.start
  constraint coincident L22 L26.end
  constraint perpendicular L22 L26
  constraint coincident L23 L27.start
  constraint coincident L17 L27.end
  constraint perpendicular L17 L27
  measures "d222" distance of L20 L26
  measures "d223" distance of L24 L27
extrude "Extrusion5" add sketch "Skizze13" along normal blind 2.25 contours L4 A2 L5 A3 L6 L20 A9 L21 L22 A10 L26 | L15 A7 L16 A8 L17 L23 A11 L24 A12 L25 L27
sketch "Skizze8" plane through (0, 0, -6.9849) normal (0, 0, -1) x (1, 0, 0)
  circle A0 centre (14.5052, -5.4485) radius 32.5
  spline S0 degree 3 poles (35.0052, 29.0515) (36.8795, 29.0515) (38.8639, 28.6884) (40.741, 27.9116) (42.1372, 27.3338) (43.4713, 26.5301) (44.6549, 25.5356) (46.3943, 24.074) (47.7962, 22.1974) (48.704, 20.1624) (49.5899, 18.1766) (50.0052, 16.0511) (50.0052, 14.0515) (50.0052, 1.0515) (50.0052, -11.9485) (50.0052, -24.9485) (50.0052, -26.8227) (49.6421, -28.8072) (48.8653, -30.6842) (48.2875, -32.0805) (47.4838, -33.4146) (46.4893, -34.5981) (45.0277, -36.3376) (43.1511, -37.7395) (41.1162, -38.6473) (39.1303, -39.5331) (37.0049, -39.9485) (35.0052, -39.9485) (21.3386, -39.9485) (7.6719, -39.9485) (-5.9948, -39.9485) (-7.869, -39.9485) (-9.8534, -39.5853) (-11.7305, -38.8085) (-13.1268, -38.2307) (-14.4609, -37.4271) (-15.6444, -36.4326) (-17.3839, -34.971) (-18.7858, -33.0943) (-19.6935, -31.0594) (-20.5794, -29.0736) (-20.9948, -26.9481) (-20.9948, -24.9485) (-20.9948, -11.9485) (-20.9948, 1.0515) (-20.9948, 14.0515) (-20.9948, 15.9258) (-20.6316, 17.9102) (-19.8548, 19.7872) (-19.277, 21.1835) (-18.4733, 22.5176) (-17.4789, 23.7011) (-16.0173, 25.4406) (-14.1406, 26.8425) (-12.1057, 27.7503) (-10.1199, 28.6362) (-7.9944, 29.0515) (-5.9948, 29.0515) (7.6719, 29.0515) (21.3386, 29.0515) (35.0052, 29.0515) knots 0 0 0 0 0.02269 0.02269 0.02269 0.039568 0.039568 0.039568 0.064375 0.064375 0.064375 0.088583 0.088583 0.088583 0.245965 0.245965 0.245965 0.268655 0.268655 0.268655 0.285533 0.285533 0.285533 0.31034 0.31034 0.31034 0.334548 0.334548 0.334548 0.5 0.5 0.5 0.52269 0.52269 0.52269 0.539568 0.539568 0.539568 0.564375 0.564375 0.564375 0.588583 0.588583 0.588583 0.745965 0.745965 0.745965 0.768655 0.768655 0.768655 0.785533 0.785533 0.785533 0.81034 0.81034 0.81034 0.834548 0.834548 0.834548 1 1 1 1
  circle A1 centre (-14.9948, 17.0515) radius 1.25
  circle A2 centre (44.0052, 17.0515) radius 1.25
  circle A3 centre (44.0052, -27.9485) radius 1.25
  circle A4 centre (-14.9948, -27.9485) radius 1.25
  line L0 (-14.9948, 17.0515) -> (44.0052, 17.0515) construction
  line L1 (-14.9948, 17.0515) -> (-14.9948, -27.9485) construction
  point P0 (14.5052, 17.0515)
  point P1 (-14.9948, -5.4485)
  dimension "d173" = 2.5
  dimension "d174" = 59
  dimension "d183" = 45
  constraint vertical A1.centre A4.centre
  constraint vertical A2.centre A3.centre
  constraint horizontal A1.centre A2.centre
  constraint horizontal A3.centre A4.centre
  constraint equal A1 A2
  constraint equal A1 A4
  constraint equal A3 A4
  constraint coincident A1.centre L0.start
  constraint coincident A2.centre L0.end
  constraint coincident A4.centre L1.end
  constraint midpoint L0 P0
  constraint vertical A0.centre P0
  constraint midpoint L1 P1
  constraint horizontal A0.centre P1
  measures "d173" diameter of A1
  measures "d174" distance of A1.centre A2.centre
  measures "d183" distance of A1.centre A4.centre
extrude "Extrusion6" cut sketch "Skizze8" against normal blind 10 contours A1 | A2 | A3 | A4
sketch "Skizze9" plane through (0, 0, 7.3701) normal (0, 0, 1) x (-1, 0, 0)
  arc A0 (-6.4052, 20.1382) -> (-7.4052, 19.1382) centre (-6.4052, 19.1382) ccw
  line L0 (-7.4052, 19.1382) -> (-7.4052, 11.1382)
  arc A1 (-7.4052, 11.1382) -> (-6.4052, 10.1382) centre (-6.4052, 11.1382) ccw
  line L1 (-6.4052, 10.1382) -> (13.5948, 10.1382)
  line L2 (13.5948, 20.8882) -> (13.5948, 20.1382)
  line L3 (13.5948, 9.3882) -> (-6.4052, 9.3882)
  arc A2 (-8.1552, 11.1382) -> (-6.4052, 9.3882) centre (-6.4052, 11.1382) ccw
  line L4 (-8.1552, 11.1382) -> (-8.1552, 19.1382)
  arc A3 (-6.4052, 20.8882) -> (-8.1552, 19.1382) centre (-6.4052, 19.1382) ccw
  line L5 (-6.4052, 20.8882) -> (13.5948, 20.8882)
  line L6 (13.5948, 20.1382) -> (-6.4052, 20.1382)
  line L7 (-10.1052, 11.1382) -> (-10.1052, 19.1382)
  arc A4 (-10.1052, 19.1382) -> (-11.1052, 20.1382) centre (-11.1052, 19.1382) ccw
  line L8 (-11.1052, 20.1382) -> (-31.1052, 20.1382)
  line L9 (-31.1052, 9.3882) -> (-31.1052, 10.1382)
  line L10 (-31.1052, 20.8882) -> (-11.1052, 20.8882)
  arc A5 (-9.3552, 19.1382) -> (-11.1052, 20.8882) centre (-11.1052, 19.1382) ccw
  line L11 (-9.3552, 19.1382) -> (-9.3552, 11.1382)
  arc A6 (-11.1052, 9.3882) -> (-9.3552, 11.1382) centre (-11.1052, 11.1382) ccw
  line L12 (-11.1052, 9.3882) -> (-31.1052, 9.3882)
  line L13 (-31.1052, 10.1382) -> (-11.1052, 10.1382)
  arc A7 (-11.1052, 10.1382) -> (-10.1052, 11.1382) centre (-11.1052, 11.1382) ccw
  line L14 (-28.5702, 1.4032) -> (-28.5702, -16.8468)
  line L15 (-28.5702, -16.8468) -> (-42.1202, -16.8468)
  line L16 (-42.1202, -16.8468) -> (-42.1202, 1.4032)
  line L17 (-42.1202, 1.4032) -> (-28.5702, 1.4032)
  spline S0 degree 3 poles (-35.0052, 27.0515) (-36.7488, 27.0515) (-38.4915, 26.6961) (-40.0958, 26.0134) (-41.2892, 25.5055) (-42.4058, 24.8178) (-43.3964, 23.9807) (-44.8523, 22.7503) (-46.0324, 21.1954) (-46.8257, 19.4622) (-47.6, 17.7708) (-48.0052, 15.9117) (-48.0052, 14.0515) (-48.0052, 1.9582) (-48.0052, -12.8552) (-48.0052, -24.9485) (-48.0052, -26.692) (-47.6498, -28.4348) (-46.9671, -30.0391) (-46.4592, -31.2324) (-45.7716, -32.3491) (-44.9344, -33.3396) (-43.704, -34.7955) (-42.1491, -35.9756) (-40.4159, -36.769) (-38.7245, -37.5432) (-36.8654, -37.9485) (-35.0052, -37.9485) (-22.2917, -37.9485) (-6.7187, -37.9485) (5.9948, -37.9485) (7.7383, -37.9485) (9.481, -37.5931) (11.0853, -36.9103) (12.2787, -36.4025) (13.3953, -35.7148) (14.3859, -34.8777) (15.8418, -33.6473) (17.0219, -32.0924) (17.8153, -30.3592) (18.5895, -28.6678) (18.9948, -26.8087) (18.9948, -24.9485) (18.9948, -12.8552) (18.9948, 1.9582) (18.9948, 14.0515) (18.9948, 15.795) (18.6394, 17.5378) (17.9566, 19.1421) (17.4488, 20.3354) (16.7611, 21.4521) (15.924, 22.4427) (14.6936, 23.8986) (13.1387, 25.0787) (11.4054, 25.872) (9.7141, 26.6462) (7.8549, 27.0515) (5.9948, 27.0515) (-6.7187, 27.0515) (-22.2917, 27.0515) (-35.0052, 27.0515) knots 0 0 0 0 0.02269 0.02269 0.02269 0.039568 0.039568 0.039568 0.064375 0.064375 0.064375 0.088583 0.088583 0.088583 0.245965 0.245965 0.245965 0.268655 0.268655 0.268655 0.285533 0.285533 0.285533 0.31034 0.31034 0.31034 0.334548 0.334548 0.334548 0.5 0.5 0.5 0.52269 0.52269 0.52269 0.539568 0.539568 0.539568 0.564375 0.564375 0.564375 0.588583 0.588583 0.588583 0.745965 0.745965 0.745965 0.768655 0.768655 0.768655 0.785533 0.785533 0.785533 0.81034 0.81034 0.81034 0.834548 0.834548 0.834548 1 1 1 1
  line L18 (-18.2552, 11.6382) -> (-25.2552, 11.6382)
  line L19 (-25.2552, 11.6382) -> (-25.2552, 18.6382)
  line L20 (-25.2552, 18.6382) -> (-18.2552, 18.6382)
  line L21 (-18.2552, 18.6382) -> (-18.2552, 11.6382)
  line L22 (-11.6052, 11.6382) -> (-11.6052, 18.6382)
  line L23 (-11.6052, 18.6382) -> (-16.6052, 15.1382)
  line L24 (-16.6052, 15.1382) -> (-11.6052, 11.6382)
  line L25 (1.0948, 13.3882) -> (1.0948, 16.8882)
  line L26 (1.0948, 16.8882) -> (-0.6552, 16.8882)
  line L27 (-0.6552, 16.8882) -> (-0.6552, 18.6382)
  line L28 (-0.6552, 18.6382) -> (-4.1552, 18.6382)
  line L29 (-4.1552, 18.6382) -> (-4.1552, 16.8882)
  line L30 (-4.1552, 16.8882) -> (-5.9052, 16.8882)
  line L31 (-5.9052, 16.8882) -> (-5.9052, 13.3882)
  line L32 (-5.9052, 13.3882) -> (-4.1552, 13.3882)
  line L33 (-4.1552, 13.3882) -> (-4.1552, 11.6382)
  line L34 (-4.1552, 11.6382) -> (-0.6552, 11.6382)
  line L35 (-0.6552, 11.6382) -> (-0.6552, 13.3882)
  line L36 (-0.6552, 13.3882) -> (1.0948, 13.3882)
  line L37 (13.5948, 10.1382) -> (13.5948, 9.3882)
  line L38 (-31.1052, 20.1382) -> (-31.1052, 20.8882)
  dimension "d184" = 1.5
  dimension "d185" = 1.5
  dimension "d186" = 1.5
  dimension "d187" = 5
  dimension "d188" = 1.65
  dimension "d189" = 1.5
  dimension "d190" = 1.5
  dimension "d191" = 1.5
  dimension "d192" = 1.75
  constraint horizontal L18
  constraint vertical L19
  constraint horizontal L20
  constraint vertical L21
  constraint vertical L22
  constraint equal L23 L24
  constraint horizontal L18.start L22.start
  constraint horizontal L20.end L22.end
  constraint equal L18 L21
  constraint perpendicular L1 L25
  constraint perpendicular L25 L26
  constraint perpendicular L26 L27
  constraint perpendicular L27 L28
  constraint perpendicular L28 L29
  constraint perpendicular L27 L30
  constraint perpendicular L28 L31
  constraint perpendicular L27 L32
  constraint perpendicular L32 L33
  constraint perpendicular L33 L34
  constraint perpendicular L34 L35
  constraint perpendicular L35 L36
  constraint horizontal L32.end L35.end
  constraint horizontal L26.end L29.end
  constraint vertical L29.end L32.end
  constraint vertical L26.end L35.end
  constraint equal L35 L36
  constraint equal L26 L27
  constraint equal L29 L30
  constraint equal L31 L34
  measures "d184" distance of L13 L22.start
  measures "d185" distance of L8 L22.end
  measures "d186" distance of L7 L22
  measures "d187" distance of L22 L23.end
  measures "d188" distance of L21 L23.end
  measures "d189" distance of L1 L34
  measures "d190" distance of L6 L28
  measures "d191" distance of L0 L31
  measures "d192" distance of L32.end L33.end
extrude "Extrusion7" cut sketch "Skizze9" against normal blind 0.75 contours L18 L19 L20 L21 | L22 L23 L24 | L25 L26 L27 L28 L29 L30 L31 L32 L33 L34 L35 L36
chamfer "Fase1" distance 1 angle 45 4 edges at (28.5702, 7.7218, 7.3701) (35.3452, 16.8468, 7.3701) (42.1202, 7.7218, 7.3701) (35.3452, -1.4032, 7.3701)
chamfer "Fase2" distance 1 angle 45 1 edges at (-5.9948, 37.9485, 7.3701)
chamfer "Fase3" distance 6 angle 45 1 edges at (-9.5914, -16.3598, 3.5151)
sketch "Skizze14" plane through (0, 0, 5.0151) normal (0, 0, -1) x (1, 0, 0)
  line L0 (20.1052, 20.1382) -> (20.1052, 10.1382)
  line L1 (20.1052, 10.1382) -> (31.1052, 10.1382)
  line L2 (31.1052, 10.1382) -> (31.1052, 9.3882)
  line L3 (31.1052, 9.3882) -> (11.1052, 9.3882)
  arc A0 (9.3552, 11.1382) -> (11.1052, 9.3882) centre (11.1052, 11.1382) ccw
  line L4 (9.3552, 11.1382) -> (9.3552, 19.1382)
  arc A1 (11.1052, 20.8882) -> (9.3552, 19.1382) centre (11.1052, 19.1382) ccw
  line L5 (11.1052, 20.8882) -> (31.1052, 20.8882)
  line L6 (31.1052, 20.8882) -> (31.1052, 20.1382)
  line L7 (31.1052, 20.1382) -> (20.1052, 20.1382)
  line L8 (28.5702, -16.8468) -> (28.5702, 1.4032)
  line L9 (28.5702, 1.4032) -> (42.1202, 1.4032)
  line L10 (42.1202, 1.4032) -> (42.1202, -16.8468)
  line L11 (42.1202, -16.8468) -> (28.5702, -16.8468)
  line L12 (-2.5948, 10.1382) -> (-2.5948, 20.1382)
  line L13 (-2.5948, 20.1382) -> (-13.5948, 20.1382)
  line L14 (-13.5948, 20.1382) -> (-13.5948, 10.8806)
  arc A2 (-13.5948, 10.8806) -> (-4.5376, 20.8882) centre (14.5052, -5.4485) ccw
  line L15 (-4.5376, 20.8882) -> (6.4052, 20.8882)
  arc A3 (8.1552, 19.1382) -> (6.4052, 20.8882) centre (6.4052, 19.1382) ccw
  line L16 (8.1552, 19.1382) -> (8.1552, 11.1382)
  arc A4 (6.4052, 9.3882) -> (8.1552, 11.1382) centre (6.4052, 11.1382) ccw
  line L17 (6.4052, 9.3882) -> (-13.5948, 9.3882)
  line L18 (-13.5948, 9.3882) -> (-13.5948, 10.1382)
  line L19 (-13.5948, 10.1382) -> (-2.5948, 10.1382)
  line L20 (43.6202, -18.3468) -> (27.0702, -18.3468)
  line L21 (27.0702, -18.3468) -> (27.0702, 2.9032)
  line L22 (27.0702, 2.9032) -> (43.6202, 2.9032)
  line L23 (43.6202, 2.9032) -> (43.6202, -18.3468)
  dimension "d251" = -1.5
extrude "Extrusion12" add sketch "Skizze14" along normal blind 6 contours L20 L21 L22 L23
equation "d141 = d140"
equation "d145 = d144"
equation "d146 = d144"
equation "d147 = d144"
equation "d155 = d154"
equation "d158 = d154"
equation "d159 = d154"
equation "d160 = d157"
equation "d168 = d167"
equation "d185 = d184"
equation "d186 = d184"
equation "d190 = d189"
equation "d191 = d189"
equation "d209 = d208"
equation "d211 = d210 / 2"
equation "d223 = d222"
